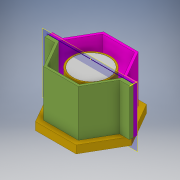
# Autodesk Inventor part: pot2
Saved by Autodesk Inventor 2019 (Build 230136000, 136)
## iProperties
Created: 2019-11-02
Part Number: pot2
Material: Generic
Document SubType Name: Modeling
Designer: assman
Density: 1 g/cm^3
Appearance: Default
Author: assman
## iProperties of the stored document pot2_3DPrint.ipt
Created: 2019-11-02
Part Number: pot2_3DPrint
Material: Generic
Document SubType Name: Modeling
Designer: assman
Density: 1 g/cm^3
Appearance: Default
Author: assman
Autodesk Inventor part; units mm, degrees
ref_plane "YZ Plane" through (0, 0, 0) normal (1, 0, 0) x (0, 1, 0)
ref_plane "XZ Plane" through (0, 0, 0) normal (0, 1, 0) x (-1, 0, 0)
ref_plane "XY Plane" through (0, 0, 0) normal (0, 0, 1) x (1, 0, 0)
sketch "Sketch1" plane through (0, 0, 0) normal (0, 1, 0) x (-1, 0, 0)
  circle A0 centre (0, 0) radius 35
  line L0 (-35, 0) -> (-17.5, 30.3109)
  line L1 (-17.5, 30.3109) -> (17.5, 30.3109)
  line L2 (17.5, 30.3109) -> (35, 0)
  line L3 (35, 0) -> (17.5, -30.3109)
  line L4 (17.5, -30.3109) -> (-17.5, -30.3109)
  line L5 (-17.5, -30.3109) -> (-35, 0)
  dimension "d0" = 70
  constraints: 12 end point, 2 coincident, 1 horizontal alignment, 15 other
extrude "Extrusion1" add sketch "Sketch1" along normal blind 10 contours L3 L4 L5 L0 L1 L2
sketch "Sketch2" plane through (0, 10, 0) normal (0, 1, 0) x (1, 0, 0)
  circle A0 centre (0, 0) radius 25
  dimension "d3" = 50
  constraints: 1 centre point, 1 coincident
  measures "d3" diameter of A0
extrude "Extrusion2" add sketch "Sketch2" along normal blind 51
sketch "Sketch3" plane through (0, 0, 0) normal (0, -1, 0) x (1, 0, 0)
  circle A0 centre (0, 0) radius 25 projected
  circle A1 centre (0, 0) radius 23
  dimension "d6" = 2
  constraints: 1 centre point
  measures "d6" radial gap between concentric circles of A0 A1
extrude "Extrusion3" cut sketch "Sketch3" against normal blind 58 contours A1
thicken "Thicken1" operation add thickness 10 both sides no extend neighbours yes toward (0, 0, 1) faces at (5.8333, 3.3333, 30.3109) (29.1667, 3.3333, 10.1036) (23.3333, 3.3333, -20.2073) (-5.8333, 3.3333, -30.3109) (-29.1667, 3.3333, -10.1036) (-23.3333, 3.3333, 20.2073)
sketch "Sketch5" plane through (0, 10, 0) normal (0, 1, 0) x (1, 0, 0)
  line L0 (41.1694, 0) -> (20.5847, -35.6538)
  line L1 (20.5847, -35.6538) -> (-20.5847, -35.6538)
  line L2 (-20.5847, -35.6538) -> (-41.1694, 0)
  line L3 (-41.1694, 0) -> (-20.5847, 35.6538)
  line L4 (-20.5847, 35.6538) -> (20.5847, 35.6538)
  line L5 (20.5847, 35.6538) -> (41.1694, 0)
  line L6 (-44.6335, 0) -> (-22.3168, -38.6538)
  line L7 (-22.3168, -38.6538) -> (22.3168, -38.6538)
  line L8 (22.3168, -38.6538) -> (44.6335, 0)
  line L9 (44.6335, 0) -> (22.3168, 38.6538)
  line L10 (22.3168, 38.6538) -> (-22.3168, 38.6538)
  line L11 (-22.3168, 38.6538) -> (-44.6335, 0)
  point P0 (0, 0)
  point P1 (0, 0)
  dimension "d12" = 3
  constraints: 24 end point, 1 coincident, 18 other
  measures "d12" distance between parallel lines of L2 L6
thicken "Thicken2" operation add thickness 5 both sides no extend neighbours yes toward (0.8660254, 0, 0.5) faces at (38.7892, 3.3333, 13.437) (31.0313, 3.3333, -26.8739) (-7.7578, 3.3333, -40.3109) (-38.7892, 6.6667, -13.437) (-31.0313, 3.3333, 26.8739) (7.7578, 6.6667, 40.3109)
extrude "Extrusion4" add sketch "Sketch5" along normal blind 60 separate body
sketch "Sketch6" plane through (0, 10, 0) normal (0, -1, 0) x (1, 0, 0)
  line L0 (-22.3168, -38.6538) -> (-44.6335, 0) projected
  line L1 (22.3168, -38.6538) -> (-22.3168, -38.6538) projected
  line L2 (44.6335, 0) -> (22.3168, -38.6538) projected
  line L3 (22.3168, 38.6538) -> (44.6335, 0) projected
  line L4 (-22.3168, 38.6538) -> (22.3168, 38.6538) projected
  line L5 (-44.6335, 0) -> (-22.3168, 38.6538) projected
  point P0 (0, 0)
extrude "Extrusion5" add sketch "Sketch6" against normal blind 3 bodies 2
sketch "Sketch7" plane through (0, 10, 0) normal (0, -1, 0) x (1, 0, 0)
  circle A0 centre (0, 0) radius 25.1
  dimension "d19" = 50.2
  constraints: 1 centre point, 1 coincident
  measures "d19" diameter of A0
extrude "Extrusion6" cut sketch "Sketch7" against normal blind 3 bodies 2
sketch "Sketch9" plane through (0, 70, 0) normal (0, 1, 0) x (1, 0, 0)
  line L0 (44.6335, 0) -> (54.6335, 0) construction
  line L1 (54.6335, 0) -> (54.6335, -5)
  line L2 (54.6335, -5) -> (54.6335, 0)
  line L3 (54.6335, 0) -> (54.6335, 5)
  line L4 (54.6335, 5) -> (41.7468, 5)
  line L5 (44.6335, 0) -> (22.3168, 38.6538) projected
  line L6 (41.7468, 5) -> (44.6335, 0)
  line L7 (44.6335, 0) -> (41.7468, -5)
  line L8 (41.7468, -5) -> (54.6335, -5)
  line L9 (0, -48.2247) -> (0, 55.3448) construction
  point P0 (0, 0)
  dimension "d22" = 10
  dimension "d23" = 5
  dimension "d24" = 5
  constraints: 18 end point, 2 collinear, 2 horizontal, 2 vertical, 1 parallel, 1 point on line
  measures "d22" distance of L0.start L0.end
  measures "d23" distance of L0.end L1.end
  measures "d24" distance of L0.end L3.end
extrude "Extrusion7" add sketch "Sketch9" against normal up to surface (60 mm away) bodies 2
mirror "Mirror1" about plane through (0, 0, 0) normal (1, 0, 0) of "Extrusion7" bodies 2
sketch "Sketch10" plane through (0, 70, 0) normal (0, 1, 0) x (1, 0, 0)
  line L0 (54.6335, -5) -> (54.6335, 5) projected
  line L1 (54.6335, 0) -> (-57.0954, 0)
  point P0 (0, 0)
  constraints: 2 end point, 1 horizontal, 1 midpoint
ref_plane "Work Plane1" through (54.6335, 70, 0) normal (0, 0, -1) x (-1, 0, 0)
split body "Split1" result two bodies by plane through (54.6335, 70, 0) normal (0, 0, -1) bodies 2 first body at (7.4389, 30, -38.1538)
sketch "Sketch11" plane through (0, 58, 0) normal (0, -1, 0) x (1, 0, 0)
  circle A0 centre (0, 0) radius 23 projected
extrude "Extrusion8" cut sketch "Sketch11" against normal blind 10 bodies 1
sketch "Sketch12" plane through (0, 61, 0) normal (0, 1, 0) x (1, 0, 0)
  circle A0 centre (0, 0) radius 25 construction
  circle A1 centre (0, 0) radius 22.9
  dimension "d30" = 45.8
  constraints: 1 centre point, 1 coincident
  measures "d30" diameter of A1
extrude "Extrusion9" add sketch "Sketch12" against normal blind 10 separate body
sketch "Sketch13" plane through (0, 51, 0) normal (0, -1, 0) x (1, 0, 0)
  circle A0 centre (0, 0) radius 22.9 projected
  circle A1 centre (0, 0) radius 20.9
  dimension "d33" = 2
  constraints: 1 centre point
  measures "d33" radial gap between concentric circles of A0 A1
extrude "Extrusion10" cut sketch "Sketch13" against normal blind 8 contours A1 bodies 5
body "Solid1"
body "Solid5"
body "Solid3"
body "Solid4"
